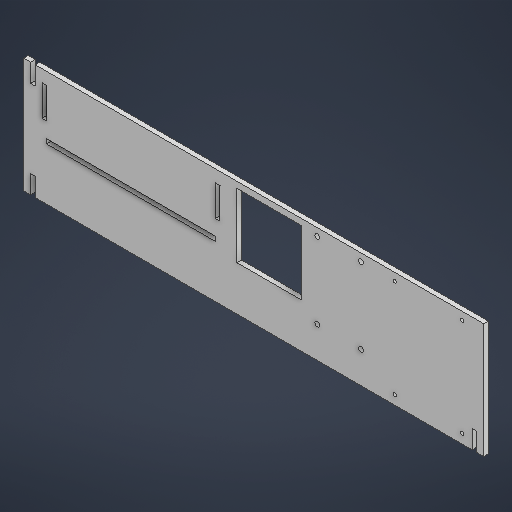
# Autodesk Inventor part: 2ndSideboard
Saved by Autodesk Inventor 2027 (Build 310192000, 192)
## iProperties
Created: 2026-06-01
Part Number: 2ndSideboard
Material: Generic
Document SubType Name: Modeling
Designer: alexy
Density: 1 g/cm^3
Appearance: Default
Author: alexy
Autodesk Inventor part; units mm, degrees
ref_plane "YZ Plane" through (0, 0, 0) normal (1, 0, 0) x (0, 1, 0)
ref_plane "XZ Plane" through (0, 0, 0) normal (0, 1, 0) x (-1, 0, 0)
ref_plane "XY Plane" through (0, 0, 0) normal (0, 0, 1) x (1, 0, 0)
sketch "Sketch1" plane through (0, 0, 0) normal (0, 0, 1) x (1, 0, 0)
  line L0 (0, 0) -> (300, 0)
  line L1 (300, 0) -> (300, 65)
  line L2 (300, 65) -> (0, 65)
  line L3 (0, 65) -> (0, 0)
  line L4 (0, 0) -> (300, 0)
  line L5 (300, 0) -> (300, -10)
  line L6 (300, -10) -> (0, -10)
  line L7 (0, -10) -> (0, 0)
  dimension "d0" = 300
  dimension "d1" = 65
  dimension "d2" = 10
  constraints: 16 end point, 4 parallel, 2 horizontal, 2 perpendicular, 1 vertical alignment
  measures "d0" distance of L1.end L2.end
  measures "d1" distance of L0.end L1.end
  measures "d2" distance of L4.end L5.end
extrude "Extrusion1" add sketch "Sketch1" along normal blind 3
sketch "Sketch3" plane through (0, 0, 3) normal (0, 0, 1) x (1, 0, 0)
  line L0 (139, 61) -> (181, 61)
  line L1 (181, 61) -> (181, 19)
  line L2 (181, 19) -> (139, 19)
  line L3 (139, 19) -> (139, 61)
  line L4 (139, 61) -> (181, 19) construction
  line L5 (181, 61) -> (139, 19) construction
  line L6 (300, -10) -> (300, 65) projected
  line L7 (300, 65) -> (0, 65) projected
  line L8 (0, 65) -> (0, -10) projected
  point P0 (0, 0)
  point P1 (160, 40)
  dimension "d12" = 25
  dimension "d13" = 42
  dimension "d14" = 42
  dimension "d19" = 160
  constraints: 12 end point, 2 midpoint, 2 parallel, 1 horizontal, 1 perpendicular
  measures "d12" distance from line of L7 point (160, 40)
  measures "d13" distance of L0.end L1.end
  measures "d14" distance of L1.end L2.end
  measures "d19" distance from line of L8 point (160, 40)
extrude "Extrusion2" cut sketch "Sketch3" against normal blind 3
sketch "Sketch2" plane through (0, 0, 3) normal (0, 0, 1) x (1, 0, 0)
  line L0 (0, -10) -> (300, -10) projected
  line L1 (4.5, -10) -> (7.5, -10)
  line L2 (7.5, -10) -> (7.5, 2)
  line L3 (7.5, 2) -> (4.5, 2)
  line L4 (4.5, 2) -> (4.5, -10)
  line L5 (295.5, -10) -> (292.5, -10)
  line L6 (292.5, -10) -> (292.5, 2)
  line L7 (292.5, 2) -> (295.5, 2)
  line L8 (295.5, 2) -> (295.5, -10)
  line L9 (300, 65) -> (0, 65) projected
  line L10 (4.5, 65) -> (7.5, 65)
  line L11 (7.5, 65) -> (7.5, 53)
  line L12 (7.5, 53) -> (4.5, 53)
  line L13 (4.5, 53) -> (4.5, 65)
  line L14 (0, 65) -> (0, -10) projected
  point P0 (0, 0)
  point P1 (294, 2)
  dimension "d5" = 4.5
  dimension "d6" = 12
  dimension "d7" = 3
  dimension "d8" = 6
  dimension "d9" = 3
  dimension "d53" = 12
  dimension "d54" = 3
  dimension "d55" = 4.5
  constraints: 24 end point, 6 parallel, 3 horizontal, 3 perpendicular, 3 point on line, 1 horizontal alignment, 1 midpoint
  measures "d5" distance of L0.start L1.start
  measures "d6" distance of L1.end L2.end
  measures "d7" distance of L1.start L1.end
  measures "d8" horizontal distance of L0.end point (294, 2)
  measures "d9" distance between parallel lines of L6 L8
  measures "d53" distance of L10.end L11.end
  measures "d54" distance of L11.end L12.end
  measures "d55" distance between parallel lines of L14 L13
extrude "Extrusion3" cut sketch "Sketch2" against normal blind 3
sketch "Sketch4" plane through (0, 0, 3) normal (0, 0, 1) x (1, 0, 0)
  line L0 (15, 27) -> (125, 27)
  line L1 (125, 27) -> (125, 24)
  line L2 (125, 24) -> (15, 24)
  line L3 (15, 24) -> (15, 27)
  line L4 (12, 57) -> (15, 57)
  line L5 (15, 57) -> (15, 37)
  line L6 (15, 37) -> (12, 37)
  line L7 (12, 37) -> (12, 57)
  line L8 (125, 57) -> (128, 57)
  line L9 (128, 57) -> (128, 37)
  line L10 (128, 37) -> (125, 37)
  line L11 (125, 37) -> (125, 57)
  line L12 (0, 65) -> (0, -10) projected
  point P0 (0, 0)
  point P1 (139, 19)
  dimension "d20" = 110
  dimension "d21" = 3
  dimension "d22" = 3
  dimension "d23" = 20
  dimension "d24" = 20
  dimension "d25" = 3
  dimension "d27" = 10
  dimension "d28" = 12
  dimension "d52" = 5
  constraints: 24 end point, 6 parallel, 3 horizontal, 3 perpendicular, 2 vertical alignment, 1 horizontal alignment
  measures "d20" distance of L1.end L2.end
  measures "d21" distance of L0.end L1.end
  measures "d22" distance of L4.start L4.end
  measures "d23" distance of L6.end L4.start
  measures "d24" distance of L8.end L9.end
  measures "d25" distance of L9.end L10.end
  measures "d27" distance of L0.end L10.end
  measures "d28" distance from line of L12 L4.start
  measures "d52" vertical distance of point (139, 19) L1.end
extrude "Extrusion4" cut sketch "Sketch4" against normal blind 3
sketch "Sketch5" plane through (0, 0, 3) normal (0, 0, 1) x (1, 0, 0)
  circle A0 centre (191.5, 60) radius 1.55
  circle A1 centre (220, 60) radius 1.55
  circle A2 centre (220, 10.5) radius 1.55
  circle A3 centre (191.5, 10.5) radius 1.55
  line L0 (300, -10) -> (300, 65) projected
  point P0 (0, 0)
  dimension "d31" = 28.5
  dimension "d32" = 49.5
  dimension "d33" = 3.1
  dimension "d34" = 3.1
  dimension "d35" = 3.1
  dimension "d36" = 3.1
  dimension "d37" = 80
  dimension "d38" = 5
  constraints: 4 centre point, 2 horizontal alignment, 2 vertical alignment
  measures "d31" distance of A1.centre A0.centre
  measures "d32" distance of A2.centre A1.centre
  measures "d33" diameter of A0
  measures "d34" diameter of A1
  measures "d35" diameter of A2
  measures "d36" diameter of A3
  measures "d37" distance from line of L0 A1.centre
  measures "d38" vertical distance of L0.end A1.centre
extrude "Extrusion5" cut sketch "Sketch5" against normal blind 3
sketch "Sketch6" plane through (0, 0, 3) normal (0, 0, 1) x (1, 0, 0)
  circle A0 centre (242, 60) radius 1.1
  circle A1 centre (286, 60) radius 1.1
  circle A2 centre (286, -4) radius 1.1
  circle A3 centre (242, -4) radius 1.1
  circle A4 centre (220, 60) radius 1.55 projected
  point P0 (0, 0)
  point P1 (300, 65)
  dimension "d41" = 2.2
  dimension "d42" = 2.2
  dimension "d43" = 2.2
  dimension "d44" = 2.2
  dimension "d45" = 64
  dimension "d46" = 44
  dimension "d50" = 5
  dimension "d51" = 14
  constraints: 4 centre point, 2 horizontal alignment, 2 vertical alignment
  measures "d41" diameter of A0
  measures "d42" diameter of A1
  measures "d43" diameter of A2
  measures "d44" diameter of A3
  measures "d45" distance of A3.centre A0.centre
  measures "d46" distance of A0.centre A1.centre
  measures "d50" vertical distance of point (300, 65) A1.centre
  measures "d51" horizontal distance of point (300, 65) A1.centre
extrude "Extrusion6" cut sketch "Sketch6" against normal blind 3 contours A0 | A1 | A2 | A3
body "Solid1"
